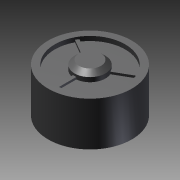
# Autodesk Inventor part: CHAMJ-E50-Rbearing
Saved by Autodesk Inventor 2015 (Build 190159000, 159)
## iProperties
Category: PARTsolutions
Company: MISUMI
Created: 2015-12-24
Part Number: CHAMJ-E50-Rbearing
Catalog Web Link: www.cadenas.de
Description: CHAMJ_E, CHAMK_E, CHAMS_Ebearing-Caster
Vendor: MISUMI
Document SubType Name: Modeling
Designer: psAdmin
Manufacturer: MISUMI
Mass: 20.6187 g
Surface Area: 53.8661 cm^2
Volume: 20.6187 cm^3
Density: 1 g/cm^3
Material: 一般
Appearance: PSOLRGB-192-192-192
PSOL_IDENT_0: {$CADENAS_DATA\23d-libs\misumi\metric\42_casters_leveling_pads\chamj_e_bearing.prj},213 {VTYP=3D},{N
PSOL_IDENT_1: B=CHAMJ-E50-Rbearing},{LINA=CHAMJ-E50-Rbearing},{NN=CHAMJ_E, CHAMK_E, CHAMS_Ebearing},{DATE=05.06.20
PSOL_IDENT_2: 15 05:25:12},{GEOMDATE=03.09.2009 00:00:00},{VERSION=},{LINEID=30},{LINESUBID=-1},{WBVAR=TSMB,MATW}
PSOL_IDENT_3: {NB=CHAMJ-E50-Rbearing},{LINA=CHAMJ-E50-Rbearing},{KT=DUMMY},{PN=CHAMJ-E50-R},{TYPE=CHAMJ-E},{TSMB=
PSOL_IDENT_4: 1},{MATMB=Low Carbon Steel},{STMB=Trivalnt Chromate},{D=50},{MATW=R},{COLORW=Black},{BSP=Available},
PSOL_IDENT_5: {BWP=Not Available},{H=65},{A=70},{C=42},{F1=56},{F2=28},{DD=6.5},{E=22},{RR=47},{B=20},{TT=2.0},{BR=
PSOL_IDENT_6: 20},{BU=21},{BN=21},{AL=300},{ALR=300},{ALU=380},{ALN=400},{MASS=180}
NN: CHAMJ_E, CHAMK_E, CHAMS_Ebearing
NT: Caster
NB: CHAMJ-E50-Rbearing
NBSYN: $PN.bearing
LINA: CHAMJ-E50-Rbearing
TSMB: Swivel
MATMB: Low Carbon Steel
STMB: Trivalnt Chromate
D: 50
MATW: Synthetic Rubber
BSP: Available
BWP: Not Available
H: 65
A: 70
C: 42
F1: 56
F2: 28
DD: 6.5
TT: 2.0
BR: 20
BU: 21
BN: 21
ALR: 300
ALU: 380
ALN: 400
SUPPLIER: MISUMI
ARTICLENO: CHAMJ-E50-Rbearing
BOMINFO: CHAMJ-E50-Rbearing
CREATOR: CADENAS GmbH
Title: CHAMJ-E50-Rbearing
Author: Cadenas PARTsolutions
Comments: Caster
Autodesk Inventor part; units mm, degrees
sketch "Sketch_1" plane through (0, 0, 0) normal (1, 0, 0) x (0, 1, 0)
  line L0 (0, -12) -> (0, 12)
  line L1 (0, 12) -> (5, 12)
  line L2 (5, 12) -> (7, 10)
  line L3 (7, 10) -> (7, 8)
  line L4 (7, 8) -> (16, 8)
  line L5 (16, 8) -> (16, 10)
  line L6 (16, 10) -> (19, 10)
  line L7 (19, 10) -> (19, -10)
  line L8 (19, -10) -> (16, -10)
  line L9 (16, -10) -> (16, -8)
  line L10 (16, -8) -> (7, -8)
  line L11 (7, -8) -> (7, -10)
  line L12 (7, -10) -> (5, -12)
  line L13 (5, -12) -> (0, -12)
  line L14 (0, -12) -> (0, 12)
  constraints: 30 end point
revolve "Revolution1" add sketch "Sketch_1" angle 360 about axis through (0, 0, -12) along (0, 0, -1)
sketch "Sketch_3" plane through (0, 0, 8) normal (0, 0, 1) x (1, 0, 0)
  line L0 (-0.75, -17) -> (0.75, -17)
  line L1 (0.75, -17) -> (0.75, -4)
  line L2 (0.75, -4) -> (-0.75, -4)
  line L3 (-0.75, -4) -> (-0.75, -17)
  constraints: 8 end point
extrude "Extrusion1" add sketch "Sketch_3" along normal blind 1
sketch "Sketch_2" plane through (0, 0, 8) normal (0, 0, 1) x (1, 0, 0)
  line L0 (3.0891, 2.6495) -> (3.8391, 1.3505)
  line L1 (3.8391, 1.3505) -> (15.0974, 7.8505)
  line L2 (15.0974, 7.8505) -> (14.3474, 9.1495)
  line L3 (14.3474, 9.1495) -> (3.0891, 2.6495)
  constraints: 8 end point
extrude "Extrusion2" add sketch "Sketch_2" along normal blind 1
sketch "Sketch_4" plane through (0, 0, 8) normal (0, 0, 1) x (1, 0, 0)
  line L0 (-15.0974, 7.8505) -> (-3.8391, 1.3505)
  line L1 (-3.8391, 1.3505) -> (-3.0891, 2.6495)
  line L2 (-3.0891, 2.6495) -> (-14.3474, 9.1495)
  line L3 (-14.3474, 9.1495) -> (-15.0974, 7.8505)
  constraints: 8 end point
extrude "Extrusion3" add sketch "Sketch_4" along normal blind 1
sketch "Sketch_5" plane through (0, 0, -8) normal (0, 0, 1) x (1, 0, 0)
  line L0 (-0.75, -17) -> (0.75, -17)
  line L1 (0.75, -17) -> (0.75, -4)
  line L2 (0.75, -4) -> (-0.75, -4)
  line L3 (-0.75, -4) -> (-0.75, -17)
  constraints: 8 end point
extrude "Extrusion4" add sketch "Sketch_5" against normal blind 1
sketch "Sketch_6" plane through (0, 0, -8) normal (0, 0, 1) x (1, 0, 0)
  line L0 (3.0891, 2.6495) -> (3.8391, 1.3505)
  line L1 (3.8391, 1.3505) -> (15.0974, 7.8505)
  line L2 (15.0974, 7.8505) -> (14.3474, 9.1495)
  line L3 (14.3474, 9.1495) -> (3.0891, 2.6495)
  constraints: 8 end point
extrude "Extrusion5" add sketch "Sketch_6" against normal blind 1
sketch "Sketch_7" plane through (0, 0, -8) normal (0, 0, 1) x (1, 0, 0)
  line L0 (-15.0974, 7.8505) -> (-3.8391, 1.3505)
  line L1 (-3.8391, 1.3505) -> (-3.0891, 2.6495)
  line L2 (-3.0891, 2.6495) -> (-14.3474, 9.1495)
  line L3 (-14.3474, 9.1495) -> (-15.0974, 7.8505)
  constraints: 8 end point
extrude "Extrusion6" add sketch "Sketch_7" against normal blind 1
ref_plane "to_wheel_XY" through (0, 0, 0) normal (0, 0, 1) x (1, 0, 0)
ref_plane "to_wheel_YZ" through (0, 0, 0) normal (1, 0, 0) x (0, 1, 0)
ref_plane "to_wheel_ZX" through (0, 0, 0) normal (0, 1, 0) x (0, 0, 1)
body "Solid1"
